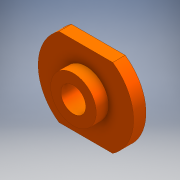
# Autodesk Inventor part: Testata Superiore
Saved by Autodesk Inventor 2016 (Build 200138000, 138)
## iProperties
Created: 2016-09-09
Part Number: Testata Superiore
Material: Generic
Document SubType Name: Modeling
Designer: Muhammad
Density: 1 g/cm^3
Appearance: Default
Author: Muhammad
Autodesk Inventor part; units mm, degrees
ref_plane "YZ Plane" through (0, 0, 0) normal (1, 0, 0) x (0, 1, 0)
ref_plane "XZ Plane" through (0, 0, 0) normal (0, 1, 0) x (-1, 0, 0)
ref_plane "XY Plane" through (0, 0, 0) normal (0, 0, 1) x (1, 0, 0)
sketch "Sketch1" plane through (0, 0, 0) normal (0, 1, 0) x (-1, 0, 0)
  line L0 (0, -19) -> (0, 19) construction
  line L1 (12.9615, 19) -> (-12.9615, 19)
  line L2 (12.9615, -19) -> (-12.9615, -19)
  arc A0 (-12.9615, 19) -> (-12.9615, -19) centre (0, 0) ccw
  arc A1 (12.9615, -19) -> (12.9615, 19) centre (0, 0) ccw
  circle A2 centre (0, 0) radius 6
  dimension "d3" = 12
  constraints: 6 end point, 4 point on circle, 3 centre point, 2 coincident, 1 horizontal, 1 parallel
  measures "d3" diameter of A2
extrude "Extrusion1" add sketch "Sketch1" along normal blind 6
sketch "Sketch2" plane through (0, 6, 0) normal (0, 1, 0) x (1, 0, 0)
  circle A0 centre (0, 0) radius 14
  dimension "d6" = 28
  constraints: 1 centre point, 1 coincident
  measures "d6" diameter of A0
extrude "Extrusion2" add sketch "Sketch2" along normal blind 4
sketch "Sketch3" plane through (0, 0, 0) normal (0, -1, 0) x (1, 0, 0)
  circle A0 centre (0, 0) radius 11
  dimension "d3" = 12
  dimension "d9" = 22
  constraints: 1 centre point, 1 coincident
  measures "d9" diameter of A0
extrude "Extrusion3" add sketch "Sketch3" along normal blind 6
sketch "Sketch4" plane through (0, -6, 0) normal (0, -1, 0) x (1, 0, 0)
  circle A0 centre (0, 0) radius 6
  constraints: 1 centre point, 1 coincident
hole "Hole1" at (0, -6, 0) direction (0, 1, 0) diameter 12 depth 11 tip angle 118
sketch "Sketch5" plane through (0, 10, 0) normal (0, 1, 0) x (1, 0, 0)
  circle A0 centre (0, 0) radius 3.25
  dimension "d19" = 6.5
  constraints: 1 centre point, 1 coincident
  measures "d19" diameter of A0
extrude "Extrusion4" cut sketch "Sketch5" against normal through all
body "Solid1"
